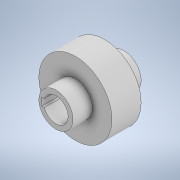
# Autodesk Inventor part: pump and e-motor coupling
Saved by Autodesk Inventor 2020 (Build 240168000, 168)
## iProperties
Created: 2020-10-19
Part Number: pump and e-motor coupling
Material: Generic
Document SubType Name: Modeling
Designer: jtri402
Density: 1 g/cm^3
Appearance: Default
Author: jtri402
Autodesk Inventor part; units mm, degrees
ref_plane "YZ Plane" through (0, 0, 0) normal (1, 0, 0) x (0, 1, 0)
ref_plane "XZ Plane" through (0, 0, 0) normal (0, 1, 0) x (-1, 0, 0)
ref_plane "XY Plane" through (0, 0, 0) normal (0, 0, 1) x (1, 0, 0)
sketch "Sketch1" plane through (0, 0, 0) normal (0, 0, 1) x (1, 0, 0)
  circle A0 centre (0, 0) radius 37.5
  dimension "d0" = 75
  constraints: 1 centre point, 1 coincident
  measures "d0" diameter of A0
extrude "Extrusion1" add sketch "Sketch1" along normal mid plane 30
sketch "Sketch2" plane through (0, 0, 15) normal (0, 0, 1) x (1, 0, 0)
  circle A0 centre (0, 0) radius 17.5
  circle A1 centre (0, 0) radius 12.5
  dimension "d3" = 35
  dimension "d4" = 25
  constraints: 2 centre point, 2 coincident
  measures "d3" diameter of A0
  measures "d4" diameter of A1
extrude "Extrusion2" add sketch "Sketch2" along normal blind 20
sketch "Sketch3" plane through (0, 0, 35) normal (0, 0, 1) x (1, 0, 0)
  line L0 (-10.5, -4) -> (-14.5, -4)
  line L1 (-14.5, -4) -> (-14.5, 4)
  line L2 (-14.5, 4) -> (-10.5, 4)
  line L3 (-10.5, 4) -> (-10.5, -4)
  circle A0 centre (0, 0) radius 12.5 projected
  line L4 (-10.5, -4) -> (-14.5, 4) construction
  line L5 (-14.5, -4) -> (-10.5, 4) construction
  point P0 (-12.5, 0)
  point P1 (-11.8427, -4)
  point P2 (-11.8427, 4)
  dimension "d7" = 4
  dimension "d8" = 8
  constraints: 12 end point, 2 midpoint, 2 parallel, 1 horizontal, 1 perpendicular, 2 other
  measures "d7" distance of L1.end L2.end
  measures "d8" distance of L0.end L1.end
extrude "Extrusion3" cut sketch "Sketch3" against normal blind 20 contours L0 L1 L2 A0
sketch "Sketch4" plane through (0, 0, -15) normal (0, 0, -1) x (-1, 0, 0)
  circle A0 centre (0, 0) radius 17.5
  circle A1 centre (0, 0) radius 4
  dimension "d11" = 8
  constraints: 2 centre point, 2 coincident
  measures "d11" diameter of A1
extrude "Extrusion4" add sketch "Sketch4" along normal blind 20
sketch "Sketch5" plane through (0, 0, -35) normal (0, 0, -1) x (-1, 0, 0)
  point P0 (0, 0)
body "Solid1"
